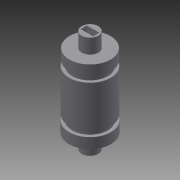
# Autodesk Inventor part: Roller
Saved by Autodesk Inventor 2015 (Build 190159000, 159)
## iProperties
Created: 2016-05-27
Part Number: Roller
Material: Generic
Document SubType Name: Modeling
Designer: Toby
Density: 1 g/cm^3
Appearance: Default
Author: Toby
Autodesk Inventor part; units mm, degrees
ref_plane "YZ Plane" through (0, 0, 0) normal (1, 0, 0) x (0, 1, 0)
ref_plane "XZ Plane" through (0, 0, 0) normal (0, 1, 0) x (-1, 0, 0)
ref_plane "XY Plane" through (0, 0, 0) normal (0, 0, 1) x (1, 0, 0)
sketch "Sketch1" plane through (0, 0, 0) normal (0, 0, 1) x (1, 0, 0)
  circle A0 centre (0, 0) radius 10
  dimension "d0" = 20
  constraints: 1 centre point, 1 coincident
  measures "d0" diameter of A0
extrude "Extrusion1" add sketch "Sketch1" along normal blind 5
sketch "Sketch2" plane through (0, 0, 5) normal (0, 0, 1) x (1, 0, 0)
  circle A0 centre (0, 0) radius 8.5
  circle A1 centre (-6.4588, 5.5258) radius 1.5
  dimension "d3" = 17
  dimension "d4" = 3
  constraints: 1 centre point, 1 coincident, 3 other
  measures "d4" diameter of A1
extrude "Extrusion2" add sketch "Sketch2" along normal blind 2.5 contours A0 A1 | A1 A0 picked at (2.8228, -1.7231) picked at (-6.0787, 5.1859)
sketch "Sketch3" plane through (0, 0, 7.5) normal (0, 0, 1) x (1, 0, 0)
  circle A0 centre (0, 0) radius 8.5 projected
  circle A1 centre (0, 8.5) radius 1.25
  dimension "d7" = 2.5
  constraints: 1 centre point, 1 vertical alignment, 1 other
  measures "d7" diameter of A1
extrude "Extrusion3" cut sketch "Sketch3" against normal blind 2.5 contours A1 A0 | A0 A1 picked at (0, 8.0765) picked at (0.0361, 8.9083)
sketch "Sketch4" plane through (0, 0, 7.5) normal (0, 0, 1) x (1, 0, 0)
  line L0 (-1.2337, 8.4081) -> (1.2466, 8.4081)
  circle A0 centre (0.0064, 8.4081) radius 0.5
  circle A1 centre (0, 0) radius 10 projected
  dimension "d10" = 8.4081
  dimension "d11" = 1
  constraints: 2 end point, 1 centre point, 1 horizontal, 1 midpoint
  measures "d10" distance of A1.centre A0.centre
  measures "d11" diameter of A0
extrude "Extrusion4" add sketch "Sketch4" against normal blind 2.5 contours A0 L0 | L0 A0
sketch "Sketch5" plane through (0, 0, 7.5) normal (0, 0, 1) x (1, 0, 0)
  circle A0 centre (0, 0) radius 9.9248
  constraints: 1 centre point, 1 coincident
extrude "Extrusion5" add sketch "Sketch5" along normal blind 20
sketch "Sketch6" plane through (0, 0, 27.5) normal (0, 0, 1) x (1, 0, 0)
  circle A0 centre (0, 0) radius 8.5
  constraints: 1 centre point, 1 coincident
extrude "Extrusion6" add sketch "Sketch6" along normal blind 2.5
sketch "Sketch7" plane through (0, 0, 30) normal (0, 0, 1) x (1, 0, 0)
  circle A0 centre (0.0064, 8.4081) radius 0.5 projected
  circle A1 centre (0.0064, 8.4081) radius 0.5
  circle A2 centre (0.0064, 8.4081) radius 1.1746
  point P0 (0, 0)
  constraints: 2 centre point, 2 coincident
extrude "Extrusion7" cut sketch "Sketch7" against normal blind 2.5 contours A0 | A2
sketch "Sketch8" plane through (0, 0, 30) normal (0, 0, 1) x (1, 0, 0)
  circle A0 centre (0.0064, 8.4081) radius 0.5 projected
  circle A1 centre (0.0064, 8.4081) radius 0.5
  point P0 (0, 0)
  constraints: 1 centre point, 1 coincident
extrude "Extrusion8" add sketch "Sketch8" against normal blind 2.5
sketch "Sketch9" plane through (0, 0, 30) normal (0, 0, 1) x (1, 0, 0)
  circle A0 centre (0, 0) radius 9.8132
  constraints: 1 centre point, 1 coincident
extrude "Extrusion9" add sketch "Sketch9" along normal blind 5
sketch "Sketch10" plane through (0, 0, 35) normal (0, 0, 1) x (1, 0, 0)
  circle A0 centre (0, 0) radius 4
  line L0 (-3, 1.5) -> (3, 1.5)
  line L1 (3, 1.5) -> (3, -1.5)
  line L2 (3, -1.5) -> (-3, -1.5)
  line L3 (-3, -1.5) -> (-3, 1.5)
  dimension "d24" = 8
  dimension "d25" = 6
  dimension "d26" = 3
  dimension "d27" = 1.5
  dimension "d28" = 3
  constraints: 8 end point, 2 parallel, 1 centre point, 1 coincident, 1 horizontal, 1 perpendicular
  measures "d24" diameter of A0
  measures "d25" distance of L0.start L0.end
  measures "d26" distance of L2.end L0.start
  measures "d27" distance from line of point (0, 0) L0
  measures "d28" distance from line of point (0, 0) L3
extrude "Extrusion10" add sketch "Sketch10" along normal blind 7
sketch "Sketch11" plane through (0, 0, 0) normal (0, 0, -1) x (-1, 0, 0)
  circle A0 centre (0, 0) radius 4
  dimension "d31" = 8
  constraints: 1 centre point, 1 coincident
  measures "d31" diameter of A0
extrude "Extrusion11" add sketch "Sketch11" along normal blind 7
body "Solid1"
